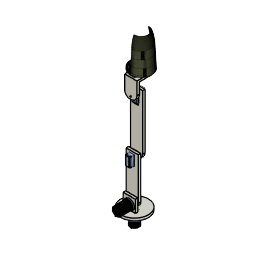
robotic arm model 2 (Autodesk Fusion 360 design; units mm, degrees)
Autodesk Fusion 360 part; units mm, degrees
sketch "Sketch1" plane through (0, 0, 0) normal (0, 0, 1) x (1, 0, 0)
sketch "Sketch2" plane through (0, 0, 0) normal (0, 0, 1) x (1, 0, 0)
  line L0 (0, 250) -> (50, 250)
  line L1 (50, 250) -> (50, 0)
  line L2 (50, 0) -> (0, 0)
  line L3 (0, 0) -> (0, 250)
  constraint horizontal L0
  constraint vertical L1
  constraint horizontal L2
  constraint vertical L3
extrude "Extrude1" add sketch "Sketch2" along normal blind 10 makes body 1
copy_body "CopyPasteBodies1" bodies 1 makes body 2
move_body "Move1" bodies 2 to x (1, 0, 0) y (0, 1, 0) z (0, 0, 1) at (80, 0, 0)
sketch "Sketch3" plane through (0, 0, 10) normal (0, 0, 1) x (-1, 0, 0)
  line L0 (-80, 0) -> (-130, 0)
  line L1 (-130, 0) -> (-130, -250)
  line L2 (-130, -250) -> (-80, -250)
  line L3 (-80, -250) -> (-80, 0)
  line L4 (-115, -10) -> (-95, -10)
  line L5 (-95, -10) -> (-95, -50)
  line L6 (-95, -50) -> (-115, -50)
  line L7 (-115, -50) -> (-115, -10)
  constraint parallel L0 L4
  constraint perpendicular L4 L5
  constraint perpendicular L5 L6
  constraint perpendicular L4 L7
extrude "Extrude2" cut sketch "Sketch3" against normal blind 10 contours L4 L5 L6 L7 bodies 2
other "Base Mesh Feature1"
other "Modify1"
sketch "Sketch4" plane through (0, 0, 10) normal (0, 0, 1) x (-1, 0, 0)
  line L0 (-95, -10) -> (-95, -50)
  line L1 (-95, -50) -> (-115, -50)
  line L2 (-115, -50) -> (-115, -10)
  line L3 (-115, -10) -> (-95, -10)
  line L4 (-80, 0) -> (-130, 0)
  line L5 (-130, 0) -> (-130, -250)
  line L6 (-130, -250) -> (-80, -250)
  line L7 (-80, -250) -> (-80, 0)
  line L8 (-130, -240) -> (-80, -240)
  line L9 (-80, -240) -> (-80, -250)
  line L10 (-80, -250) -> (-130, -250)
  line L11 (-130, -250) -> (-130, -240)
  constraint horizontal L8
  constraint vertical L9
  constraint horizontal L10
  constraint vertical L11
  constraint coincident L6.end L7.start
  constraint coincident L5 L8.start
extrude "Extrude3" add sketch "Sketch4" along normal blind 40 contours L5 L6 L7 L8 L9 L10 L11 bodies 2
sketch "Sketch5" plane through (0, 0, 10) normal (0, 0, 1) x (-1, 0, 0)
  line L0 (0, 0) -> (-50, 0)
  line L1 (-50, 0) -> (-50, -250)
  line L2 (-50, -250) -> (0, -250)
  line L3 (0, -250) -> (0, 0)
  line L4 (-35, -10) -> (-15, -10)
  line L5 (-15, -10) -> (-15, -50)
  line L6 (-15, -50) -> (-35, -50)
  line L7 (-35, -50) -> (-35, -10)
  constraint horizontal L4
  constraint vertical L5
  constraint horizontal L6
  constraint vertical L7
extrude "Extrude4" cut sketch "Sketch5" against normal blind 10 contours L4 L5 L6 L7 bodies 1
other "Modify2"
other "Modify3"
sketch "Sketch6" plane through (0, 0, 10) normal (0, 0, 1) x (-1, 0, 0)
  line L0 (-130, -240) -> (-80, -240)
  line L1 (-80, -240) -> (-80, 0)
  line L2 (-80, 0) -> (-130, 0)
  line L3 (-130, 0) -> (-130, -240)
  line L4 (-95, -10) -> (-95, -50)
  line L5 (-95, -50) -> (-115, -50)
  line L6 (-115, -50) -> (-115, -10)
  line L7 (-115, -10) -> (-95, -10)
  line L8 (-115, -10) -> (-95, -10)
  line L9 (-95, -10) -> (-95, -50)
  line L10 (-95, -50) -> (-115, -50)
  line L11 (-115, -50) -> (-115, -10)
  constraint horizontal L8
  constraint vertical L9
  constraint horizontal L10
  constraint vertical L11
  constraint coincident L4.end L5.start
  constraint coincident L6.end L7.start
extrude "Extrude5" add sketch "Sketch6" against normal blind 10 contours L4 L5 L6 L7 L8 L9 L10 L11 bodies 2
hole "Hole1" at (104.9037, 12.8046, 10) direction (0, 0, -1) diameter 4 depth 30 tip angle 118 bodies 2
move_body "Move2" bodies 2 to x (1, 0, 0) y (0, 0, -1) z (0, 1, 0) at (0, 0, 250)
ref_plane "WorkPlane1" through (0, 0, 60) normal (0, 0, 1) x (1, 0, 0)
split "Split1" by plane through (0, 0, 60) normal (0, 0, 1) bodies 2 makes body 3 at (104.9679, 10, 118.3985)
move_face "MoveFace1" by (0, 0, 40) 1 faces at (104.9679, 0, 118.3985) on bodies 3
move_body "Move3" bodies 3 to x (1, 0, 0) y (0, 1, 0) z (0, 0, 1) at (0, 10, -40)
other "Base Mesh Feature2"
sketch "Sketch7" plane through (0, 0, 0) normal (0, -1, 0) x (1, 0, 0)
  line L0 (130, 60) -> (80, 60)
  line L1 (80, 60) -> (80, 0)
  line L2 (80, 0) -> (130, 0)
  line L3 (130, 0) -> (130, 60)
  circle A0 centre (105, 30) radius 20.6155
extrude "Extrude6" cut sketch "Sketch7" against normal blind 8 contours A0 bodies 2
sketch "Sketch8" plane through (0, 8, 0) normal (0, -1, 0) x (1, 0, 0)
  circle A0 centre (105, 30) radius 20.6155
  circle A1 centre (105, 30) radius 2
  constraint concentric A0 A1
extrude "Extrude7" cut sketch "Sketch8" against normal blind 26 contours A1 bodies 2 3
other "Modify4"
other "Modify5"
sketch "Sketch9" plane through (0, 10, 0) normal (0, -1, 0) x (1, 0, 0)
  circle A0 centre (105, 30) radius 2
  line L0 (80, 20) -> (130, 20)
  line L1 (130, 20) -> (130, 210)
  line L2 (130, 210) -> (80, 210)
  line L3 (80, 210) -> (80, 20)
  circle A1 centre (104.9037, 197.1954) radius 2
  line L4 (93.2499, 200.3737) -> (112.9909, 200.3737)
  line L5 (112.9909, 200.3737) -> (112.9909, 160.3737)
  line L6 (112.9909, 160.3737) -> (93.2499, 160.3737)
  line L7 (93.2499, 160.3737) -> (93.2499, 200.3737)
  dimension "d19" = 40
  constraint horizontal L4
  constraint vertical L5
  constraint horizontal L6
  constraint vertical L7
  measures "d19" distance of L4.start L6.end
extrude "Extrude8" cut sketch "Sketch9" against normal blind 35 contours L4 L5 L6 L7 bodies 3
other "Modify6"
other "Modify7"
fillet "Fillet1" radius 20 1 edges at (80, 15, 20) on bodies 3
fillet "Fillet2" radius 20 1 edges at (130, 15, 20) on bodies 3
other "Modify8"
other "Modify9"
hole "Hole2" at (24.9437, 234.6044, 10) direction (0, 0, -1) diameter 10 depth 40 tip angle 118 bodies 1
move_body "Move4" bodies 1 to x (1, 0, 0) y (0, 0, -1) z (0, 1, 0) at (80, 34.3994, 424.3994)
move_body "Move5" bodies 1 to x (0.819152, 0, 0.573576) y (0, 1, 0) z (-0.573576, 0, 0.819152) at (127.0387, 0, -23.0913)
move_body "Move6" bodies 1 to x (0.819152, 0, -0.573576) y (0, 1, 0) z (0.573576, 0, 0.819152) at (-104.2124, 0, 0.7892)
extrude "Extrude9" add 1 faces at (94.9403, 37.7327, 323.4069) along direction (0, 0, -1) blind 40 on bodies 1 bodies 1
sketch "Sketch11" plane through (0, 44.3994, 0) normal (0, 1, 0) x (-1, 0, 0)
  circle A0 centre (-91.5507, 98.8025) radius 5
  line L0 (-66.607, 333.4069) -> (-116.607, 333.4069)
  line L1 (-116.607, 333.4069) -> (-116.607, 83.4069)
  line L2 (-116.607, 83.4069) -> (-66.607, 83.4069)
  line L3 (-66.607, 83.4069) -> (-66.607, 333.4069)
  line L4 (-116.607, 333.4069) -> (-66.607, 333.4069)
  line L5 (-66.607, 333.4069) -> (-66.607, 325.2781)
  line L6 (-66.607, 325.2781) -> (-116.607, 325.2781)
  line L7 (-116.607, 325.2781) -> (-116.607, 333.4069)
  constraint horizontal L4
  constraint vertical L5
  constraint horizontal L6
  constraint vertical L7
  constraint coincident L3 L5.end
  constraint coincident L0.end L1.start
extrude "Extrude10" add sketch "Sketch11" against normal blind 60 contours L0 L1 L3 L4 L5 L6 L7 bodies 1
sketch "Sketch12" plane through (0, 0, 333.4069) normal (0, 0, 1) x (-1, 0, 0)
  line L0 (-116.607, 15.6006) -> (-116.607, -44.3994)
  line L1 (-116.607, -44.3994) -> (-66.607, -44.3994)
  line L2 (-66.607, -44.3994) -> (-66.607, 15.6006)
  line L3 (-66.607, 15.6006) -> (-116.607, 15.6006)
  line L4 (-103, 10) -> (-83, 10)
  line L5 (-83, 10) -> (-83, -30)
  line L6 (-83, -30) -> (-103, -30)
  line L7 (-103, -30) -> (-103, 10)
  constraint horizontal L4
  constraint vertical L5
  constraint horizontal L6
  constraint vertical L7
extrude "Extrude11" cut sketch "Sketch12" against normal blind 10 contours L4 L5 L6 L7 bodies 1
other "CopyPasteMeshes1"
other "Modify10"
other "Modify11"
other "Modify12"
move_body "Move7" bodies 1 to x (1, 0, 0) y (0, 1, 0) z (0, 0, 1) at (0, 0, 100)
other "Modify13"
move_body "Move8" bodies 1 to x (1, 0, 0) y (0, 1, 0) z (0, 0, 1) at (10, 0, 0)
other "Modify14"
other "Base Mesh Feature3"
fillet "Fillet3" radius 25 1 edges at (126.607, 39.3994, 183.4069) on bodies 1
fillet "Fillet4" radius 25 1 edges at (76.607, 39.3994, 183.4069) on bodies 1
other "Modify15"
other "Modify16"
other "CopyPasteMeshes2"
other "Modify17"
other "Modify18"
sketch "Sketch13" plane through (0, 0, 10) normal (0, 0, 1) x (-1, 0, 0)
  line L0 (-80, -10) -> (-130, -10)
  line L1 (-130, -10) -> (-130, -50)
  line L2 (-130, -50) -> (-80, -50)
  line L3 (-80, -50) -> (-80, -10)
  circle A0 centre (-105, -10) radius 55.9017
  constraint midpoint L0 A0.centre
extrude "Extrude12" add sketch "Sketch13" against normal blind 10 bodies 2
other "Modify19"
other "Modify20"
sketch "Sketch14" plane through (0, 0, 0) normal (0, 0, -1) x (1, 0, 0)
  circle A0 centre (105, -10) radius 55.9017
sketch "Sketch15" plane through (0, 0, 0) normal (0, 0, -1) x (1, 0, 0)
  circle A0 centre (105, -10) radius 18.243
extrude "Extrude13" cut sketch "Sketch15" against normal blind 7 bodies 2
other "Modify21"
ref_plane "WorkPlane2" through (0, 0, 10) normal (0, 0, 1) x (1, 0, 0)
split "Split2" by plane through (0, 0, 10) normal (0, 0, 1) bodies 2 makes body 4 at (104.9502, 10, 50.6648)
move_body "Move9" bodies 4 to x (1, 0, 0) y (0, 1, 0) z (0, 0, 1) at (0, -12, 0)
hole "Hole3" at (105, 10, 10) direction (0, 0, -1) diameter 3 depth 22 tip angle 118 bodies 2
other "Modify22"
move_body "Move10" bodies 3 to x (1, 0, 0) y (0, 1, 0) z (0, 0, 1) at (0, -10, 0)
other "Modify23"
move_body "Move11" bodies 1 to x (1, 0, 0) y (0, 1, 0) z (0, 0, 1) at (1.7242, -15, -6.1933)
other "Modify24"
other "Modify25"
ref_plane "WorkPlane3" through (0, 0, 350) normal (0, 0, 1) x (1, 0, 0)
split "Split3" by plane through (0, 0, 350) normal (0, 0, 1) bodies 1 makes body 5 at (94.9979, 29.3994, 401.4757)
move_body "Move12" bodies 5 to x (1, 0, 0) y (0, 1, 0) z (0, 0, 1) at (0, -300, 0)
extrude "Extrude14" add 1 faces at (111.6645, 22.7327, 350) along direction (0, 0, 1) blind 75 on bodies 1 bodies 1
sketch "Sketch16" plane through (0, 19.3994, 0) normal (0, -1, 0) x (1, 0, 0)
  line L0 (78.3312, 425) -> (78.3312, 202.2136)
  arc A0 (78.3312, 202.2136) -> (128.3312, 202.2136) centre (103.3312, 202.2136) ccw
  line L1 (128.3312, 202.2136) -> (128.3312, 425)
  line L2 (128.3312, 425) -> (78.3312, 425)
  circle A1 centre (103.2749, 192.6092) radius 5
  line L3 (91.7439, 414.6832) -> (111.9208, 414.6832)
  line L4 (111.9208, 414.6832) -> (111.9208, 374.3486)
  line L5 (111.9208, 374.3486) -> (91.7439, 374.3486)
  line L6 (91.7439, 374.3486) -> (91.7439, 414.6832)
  constraint horizontal L3
  constraint vertical L4
  constraint horizontal L5
  constraint vertical L6
extrude "Extrude15" cut sketch "Sketch16" against normal blind 10 contours L3 L4 L5 L6 bodies 1
other "CopyPasteMeshes3"
other "Modify26"
hole "Hole4" at (104.0047, -280.6006, 360.0303) direction (0, 1, 0) diameter 3 depth 22 tip angle 118 bodies 5
hole "Hole5" at (104.0047, -280.6006, 360.0303) direction (0, 1, 0) diameter 4 depth 22 tip angle 118 bodies 5
move_body "Move13" bodies 5 to x (-0.996195, 0.087156, 0) y (-0.087156, -0.996195, 0) z (0, 0, 1) at (161.5413, -278.2543, 40)
move_body "Move14" bodies 5 to x (1, 0, 0) y (0, 1, 0) z (0, 0, 1) at (20, 0, 5)
move_body "Move15" bodies 5 to x (1, 0, 0) y (0, 1, 0) z (0, 0, 1) at (0, -5, -5)
hole "Hole6" at (101.5168, -4.6188, 400.0303) direction (0.087156, 0.996195, 0) diameter 6 depth 22 tip angle 118 bodies 5
move_body "Move16" bodies 5 to x (1, 0, 0) y (0, 1, 0) z (0, 0, 1) at (0, 0, 2)
move_body "Move17" bodies 5 to x (0.996195, 0.087156, 0) y (-0.087156, 0.996195, 0) z (0, 0, 1) at (-0.3035, -6.7617, 0)
other "Modify27"
other "Modify28"
other "Modify29"
fillet "Fillet5" radius 20.5 1 edges at (76.9031, 2.4848, 392) on bodies 5
fillet "Fillet6" radius 25.5 1 edges at (126.9031, 2.4848, 392) on bodies 5
combine "Combine1" operation add target body 4 tool bodies 2
other "Modify30"
other "MeshRepair1"
other "MeshRepair2"
named bodies: "elbow link", "base", "shoulder link", "wrist link"
